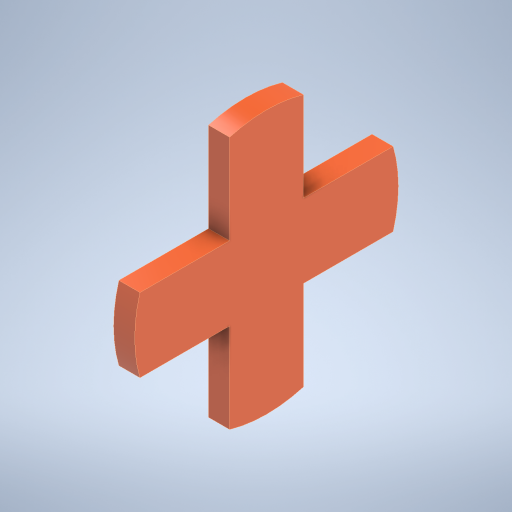
# Autodesk Inventor part: RubberSheet_1
Saved by Autodesk Inventor 2023 (Build 270158000, 158)
## iProperties
Created: 2023-10-19
Part Number: RubberSheet_1
Material: Generic
Document SubType Name: Modeling
Designer: MichihisaOohara
Density: 1 g/cm^3
Appearance: 滑らか - 淡いオレンジ
Author: MichihisaOohara
Autodesk Inventor part; units mm, degrees
ref_plane "YZ Plane" through (0, 0, 0) normal (1, 0, 0) x (0, 1, 0)
ref_plane "XZ Plane" through (0, 0, 0) normal (0, 1, 0) x (-1, 0, 0)
ref_plane "XY Plane" through (0, 0, 0) normal (0, 0, 1) x (1, 0, 0)
sketch "スケッチ1" plane through (0, 0, 0) normal (1, 0, 0) x (0, 1, 0)
  circle A0 centre (0, 0) radius 10
  circle A1 centre (0, 0) radius 12.5
  line L0 (3.5, 12.5) -> (-3.5, 12.5)
  line L1 (-3.5, 12.5) -> (-3.5, -12.5)
  line L2 (-3.5, -12.5) -> (3.5, -12.5)
  line L3 (3.5, -12.5) -> (3.5, 12.5)
  line L4 (3.5, 12.5) -> (-3.5, -12.5) construction
  line L5 (-3.5, 12.5) -> (3.5, -12.5) construction
  line L6 (-12.5, 3.5) -> (12.5, 3.5)
  line L7 (12.5, 3.5) -> (12.5, -3.5)
  line L8 (12.5, -3.5) -> (-12.5, -3.5)
  line L9 (-12.5, -3.5) -> (-12.5, 3.5)
  line L10 (-12.5, 3.5) -> (12.5, -3.5) construction
  line L11 (12.5, 3.5) -> (-12.5, -3.5) construction
  point P0 (12, -3.5)
  point P1 (12, 3.5)
  point P2 (3.5, 3.5)
  point P3 (3.5, 12)
  point P4 (-3.5, 12)
  point P5 (-3.5, 3.5)
  point P6 (-12, 3.5)
  point P7 (-12, -3.5)
  point P8 (-3.5, -3.5)
  point P9 (-3.5, -12)
  point P10 (3.5, -12)
  point P11 (3.5, -3.5)
  dimension "d0" = 20
  dimension "d1" = 25
  dimension "d2" = 7
  dimension "d3" = 25
  dimension "d4" = 25
  dimension "d5" = 7
  constraints: 24 end point, 4 midpoint, 4 parallel, 2 centre point, 2 coincident, 2 horizontal, 2 perpendicular
  measures "d0" diameter of A0
  measures "d1" diameter of A1
  measures "d2" distance of L0.start L0.end
  measures "d3" distance of L2.end L0.start
  measures "d4" distance of L6.start L6.end
  measures "d5" distance of L6.end L7.end
extrude "押し出し1" add sketch "スケッチ1" along normal blind 2 contours A0 L8 L3 L6 | A0 L6 A1 L8 | L3 L6 L1 A0 | A0 L1 A1 L3 | L3 L8 L1 L6 | L3 A1 L1 A0 | A0 L1 L8 L3 | L1 L8 A0 L6 | A0 L8 A1 L6
equation "\"d5\" = d2"
